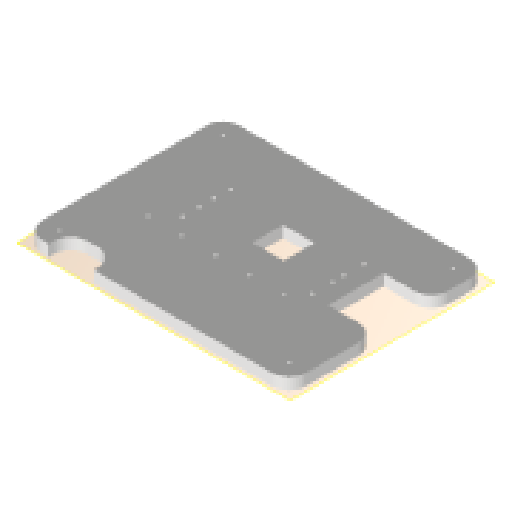
# Autodesk Inventor part: 60_Planktoscope_MicroscopeHolder_Bottom_v0
Saved by Autodesk Inventor 2024.1 (Build 281209000, 209)
## iProperties
Created: 2024-06-29
Part Number: 60_Planktoscope_MicroscopeHolder_Bottom_v0
Material: Generisch
Document SubType Name: Modeling
Designer: diederichbenedict
Density: 1 g/cm^3
Appearance: Vorgabe
Author: diederichbenedict
Autodesk Inventor part; units mm, degrees
ref_plane "YZ Plane" through (0, 0, 0) normal (1, 0, 0) x (0, 1, 0)
ref_plane "XZ Plane" through (0, 0, 0) normal (0, 1, 0) x (-1, 0, 0)
ref_plane "XY Plane" through (0, 0, 0) normal (0, 0, 1) x (1, 0, 0)
ref_plane "Arbeitsebene1" through (0, 0, -15) normal (0, 0, 1) x (1, 0, 0)
sketch "Skizze1" plane through (0, 0, -15) normal (0, 0, 1) x (1, 0, 0)
  line L0 (-108.9123, -85.8768) -> (-108, -84.9645) construction
  line L1 (-108, -84.9645) -> (-105.5687, -87.3957) construction
  arc A0 (-105.5687, -87.3957) -> (-101.5, -88) centre (-101.5, -74) ccw construction
  line L2 (-101.5, -88) -> (-95.5, -88) construction
  line L3 (-95.5, -88) -> (-95.5, -75) construction
  arc A1 (-88.5, -68) -> (-95.5, -75) centre (-88.5, -75) ccw construction
  line L4 (-88.5, -68) -> (-62.5, -68) construction
  arc A2 (-55.5, -75) -> (-62.5, -68) centre (-62.5, -75) ccw construction
  line L5 (-55.5, -75) -> (-55.5, -88) construction
  line L6 (-55.5, -88) -> (101.7625, -88) construction
  arc A3 (101.7625, -88) -> (115.5, -74) centre (101.5, -74.0025) ccw construction
  line L7 (115.5, -74) -> (115.5, 74) construction
  arc A4 (115.5, 74) -> (101.7625, 88) centre (101.5, 74.0025) ccw construction
  line L8 (101.7625, 88) -> (-101.5, 88) construction
  arc A5 (-101.5, 88) -> (-115.5, 74) centre (-101.5, 74) ccw construction
  line L9 (-115.5, 74) -> (-115.5, -74) construction
  arc A6 (-115.5, -74) -> (-108.9123, -85.8768) centre (-101.5, -74) ccw construction
  line L10 (101.6984, -82) -> (101.3016, -82) construction
  arc A7 (101.3016, -82) -> (101.6984, -82) centre (101.5, -74.0025) ccw construction
  line L11 (95.5, 73) -> (95.5, 82) construction
  arc A8 (95.5, 73) -> (100.5, 68) centre (100.5, 73) ccw construction
  line L12 (109.5, 68) -> (100.5, 68) construction
  line L13 (109.5, 68) -> (109.5, -68) construction
  line L14 (100.5, -68) -> (109.5, -68) construction
  arc A9 (100.5, -68) -> (95.5, -73) centre (100.5, -73) ccw construction
  line L15 (95.5, -82) -> (95.5, -73) construction
  line L16 (95.5, -82) -> (-49.5, -82) construction
  line L17 (-49.5, -82) -> (-49.5, -75) construction
  arc A10 (-49.5, -75) -> (-62.5, -62) centre (-62.5, -75) ccw construction
  line L18 (-62.5, -62) -> (-88.5, -62) construction
  arc A11 (-88.5, -62) -> (-99.5163, -68.0977) centre (-88.5, -75) ccw construction
  arc A12 (-99.5163, -68.0977) -> (-100.5, -68) centre (-100.5, -73) ccw construction
  line L19 (-109.5, -68) -> (-100.5, -68) construction
  line L20 (-109.5, -68) -> (-109.5, 68) construction
  line L21 (-100.5, 68) -> (-109.5, 68) construction
  arc A13 (-100.5, 68) -> (-95.5, 73) centre (-100.5, 73) ccw construction
  line L22 (-95.5, 82) -> (-95.5, 73) construction
  line L23 (-95.5, 82) -> (95.5, 82) construction
  arc A14 (101.6984, 82) -> (101.3016, 82) centre (101.5, 74.0025) ccw construction
  line L24 (101.3016, 82) -> (101.6984, 82) construction
  line L25 (111.5331, 80.5) -> (107.9975, 76.9645) construction
  line L26 (107.9975, 76.9645) -> (104.462, 80.5) construction
  line L27 (104.462, 80.5) -> (107.9975, 84.0355) construction
  line L28 (107.9975, 84.0355) -> (111.5331, 80.5) construction
  line L29 (108, -84.0355) -> (104.4645, -80.5) construction
  line L30 (104.4645, -80.5) -> (108, -76.9645) construction
  line L31 (108, -76.9645) -> (111.5355, -80.5) construction
  line L32 (111.5355, -80.5) -> (108, -84.0355) construction
  line L33 (-108, 76.9645) -> (-111.5355, 80.5) construction
  line L34 (-111.5355, 80.5) -> (-108, 84.0355) construction
  line L35 (-108, 84.0355) -> (-104.4645, 80.5) construction
  line L36 (-104.4645, 80.5) -> (-108, 76.9645) construction
  circle A15 centre (58.5, 18.7) radius 1.4 projected
  circle A16 centre (58.5, 36.552) radius 1.4 projected
  circle A17 centre (-57.5, 20.252) radius 1.4 projected
  circle A18 centre (-57.5, 35) radius 1.4 projected
  line L37 (-60.5, 13.7) -> (-60.5, 38) construction
  line L38 (61.5, 13.7) -> (-60.5, 13.7) construction
  line L39 (61.5, 38) -> (61.5, 13.7) construction
  line L40 (61.5, 38) -> (-60.5, 38) construction
  circle A19 centre (58.5, 8.7) radius 1.4 projected
  circle A20 centre (58.5, -9.152) radius 1.4 projected
  circle A21 centre (-57.5, 7.148) radius 1.4 projected
  circle A22 centre (-57.5, -7.6) radius 1.4 projected
  line L41 (-60.5, 13.7) -> (-60.5, -10.6) construction
  line L42 (61.5, -10.6) -> (-60.5, -10.6) construction
  line L43 (61.5, -10.6) -> (61.5, 13.7) construction
  line L44 (61.5, 13.7) -> (-60.5, 13.7) construction
  line L45 (-101.5, 87.5) -> (101.5, 87.5)
  line L46 (116.5, 72.5) -> (116.5, -72.3481)
  line L47 (101.5, -87.3481) -> (-101.5, -87.3481)
  line L48 (-116.5, -72.3481) -> (-116.5, 72.5)
  arc A23 (-116.5, -72.3481) -> (-101.5, -87.3481) centre (-101.5, -72.3481) ccw
  arc A24 (-101.5, 87.5) -> (-116.5, 72.5) centre (-101.5, 72.5) ccw
  arc A25 (116.5, 72.5) -> (101.5, 87.5) centre (101.5, 72.5) ccw
  arc A26 (101.5, -87.3481) -> (116.5, -72.3481) centre (101.5, -72.3481) ccw
  line L49 (-95.5, -88) -> (-56.1, -88)
  line L50 (-56.1, -88) -> (-56.1, -83)
  line L51 (-71.1, -68) -> (-80.5, -68)
  line L52 (-95.5, -83) -> (-95.5, -88)
  arc A27 (-80.5, -68) -> (-95.5, -83) centre (-80.5, -83) ccw
  arc A28 (-56.1, -83) -> (-71.1, -68) centre (-71.1, -83) ccw
  point P0 (0, 0)
  point P1 (-103.5567, -87.8481)
  point P2 (-95.5, -87.3481)
  point P3 (-56.1, -87.3481)
  dimension "d0" = 1
  dimension "d1" = 1
  dimension "d2" = 0.5
  dimension "d3" = 0.5
  dimension "d4" = 15
  dimension "d5" = 15
  constraints: 16 end point, 13 point on circle, 12 tangent, 6 centre point, 4 equal radius, 4 parallel, 2 horizontal, 2 perpendicular
  measures "d0" distance between parallel lines of L48 L9
  measures "d1" distance between parallel lines of L7 L46
  measures "d2" distance between parallel lines of L45 L8
  measures "d3" distance from line of point (-103.557, -87.848) L47
  measures "d4" radius of A23
  measures "d5" radius of A27
extrude "Extrusion1" add sketch "Skizze1" along normal blind 10 draft -1 contours L45 A25 L46 A26 L47 L50 A28 L51 A27 L52 A23 L48 A24
sketch "Skizze3" plane through (0, 0, -5) normal (0, 0, 1) x (1, 0, 0)
  line L0 (116.3254, 72.5) -> (116.3254, -72.3481) projected
  arc A0 (116.3254, 72.5) -> (101.5, 87.3254) centre (101.5, 72.5) ccw projected
  line L1 (-101.5, 87.3254) -> (101.5, 87.3254) projected
  arc A1 (-101.5, 87.3254) -> (-116.3254, 72.5) centre (-101.5, 72.5) ccw projected
  line L2 (-116.3254, -72.3481) -> (-116.3254, 72.5) projected
  arc A2 (-116.3254, -72.3481) -> (-101.5, -87.1736) centre (-101.5, -72.3481) ccw projected
  line L3 (-95.6746, -87.1736) -> (-101.5, -87.1736) projected
  line L4 (-95.6746, -83) -> (-95.6746, -87.1736) projected
  arc A3 (-80.5, -67.8254) -> (-95.6746, -83) centre (-80.5, -83) ccw projected
  line L5 (-71.1, -67.8254) -> (-80.5, -67.8254) projected
  arc A4 (-55.9254, -83) -> (-71.1, -67.8254) centre (-71.1, -83) ccw projected
  line L6 (-55.9254, -87.1736) -> (-55.9254, -83) projected
  line L7 (101.5, -87.1736) -> (-55.9254, -87.1736) projected
  arc A5 (101.5, -87.1736) -> (116.3254, -72.3481) centre (101.5, -72.3481) ccw projected
  circle A6 centre (58.5, 18.7) radius 1.5746 projected
  circle A7 centre (58.5, 36.552) radius 1.5746 projected
  circle A8 centre (-57.5, 20.252) radius 1.5746 projected
  circle A9 centre (-57.5, 35) radius 1.5746 projected
  circle A10 centre (58.5, 8.7) radius 1.5746 projected
  circle A11 centre (58.5, -9.152) radius 1.5746 projected
  circle A12 centre (-57.5, 7.148) radius 1.5746 projected
  circle A13 centre (-57.5, -7.6) radius 1.5746 projected
  point P0 (0, 0)
hole "Bohrung1" at (-101.5, 72.5, -5) at (-101.5, -72.3481, -5) at (101.5, -72.3481, -5) at (101.5, 72.5, -5) direction (0, 0, -1) diameter 2.8 end through all
sketch "Skizze4" plane through (0, 0, -5) normal (0, 0, 1) x (1, 0, 0)
  line L0 (-2.75, 38) -> (-2.75, 23.7) projected
  line L1 (-6.0553, 13.7) -> (-6.0553, 30)
  line L2 (20.9, 30.6837) -> (20.9, 6.6837) projected
  line L3 (20.9, 30.6837) -> (-6.8742, 30.6837)
  line L4 (-6.8742, 30.6837) -> (-6.8742, 3.5446)
  line L5 (-6.8742, 3.5446) -> (20.9, 3.5446)
  line L6 (20.9, 3.5446) -> (20.9, 30.6837)
  point P0 (0, 0)
  constraints: 10 end point, 2 parallel, 1 horizontal, 1 perpendicular, 1 vertical, 2 other
extrude "Extrusion3" cut sketch "Skizze4" against normal through all
sketch "Skizze5" plane through (0, 0, -5) normal (0, 0, 1) x (1, 0, 0)
  line L0 (-6.8742, 30.6837) -> (20.9, 30.6837) projected
  line L1 (20.9, 30.6837) -> (20.9, 3.5446) projected
  line L2 (20.9, 3.5446) -> (-6.8742, 3.5446) projected
  line L3 (-6.8742, 3.5446) -> (-6.8742, 30.6837) projected
  circle A0 centre (101.5, 72.5) radius 1.4 projected
  circle A1 centre (101.5, -72.3481) radius 1.4 projected
  circle A2 centre (-101.5, -72.3481) radius 1.4 projected
  circle A3 centre (-101.5, 72.5) radius 1.4 projected
  line L4 (116.3254, 72.5) -> (116.3254, -72.3481) projected
  arc A4 (116.3254, 72.5) -> (101.5, 87.3254) centre (101.5, 72.5) ccw projected
  line L5 (-101.5, 87.3254) -> (101.5, 87.3254) projected
  arc A5 (-101.5, 87.3254) -> (-116.3254, 72.5) centre (-101.5, 72.5) ccw projected
  line L6 (-116.3254, -72.3481) -> (-116.3254, 72.5) projected
  arc A6 (-116.3254, -72.3481) -> (-101.5, -87.1736) centre (-101.5, -72.3481) ccw projected
  line L7 (-95.6746, -87.1736) -> (-101.5, -87.1736) projected
  line L8 (-95.6746, -83) -> (-95.6746, -87.1736) projected
  arc A7 (-80.5, -67.8254) -> (-95.6746, -83) centre (-80.5, -83) ccw projected
  line L9 (-71.1, -67.8254) -> (-80.5, -67.8254) projected
  arc A8 (-55.9254, -83) -> (-71.1, -67.8254) centre (-71.1, -83) ccw projected
  line L10 (-55.9254, -87.1736) -> (-55.9254, -83) projected
  line L11 (101.5, -87.1736) -> (-55.9254, -87.1736) projected
  arc A9 (101.5, -87.1736) -> (116.3254, -72.3481) centre (101.5, -72.3481) ccw projected
  circle A10 centre (58.5, 18.7) radius 1.5746 projected
  circle A11 centre (58.5, 36.552) radius 1.5746 projected
  circle A12 centre (-57.5, 20.252) radius 1.5746 projected
  circle A13 centre (-57.5, 35) radius 1.5746 projected
  circle A14 centre (58.5, 8.7) radius 1.5746 projected
  circle A15 centre (58.5, -9.152) radius 1.5746 projected
  circle A16 centre (-57.5, 7.148) radius 1.5746 projected
  circle A17 centre (-57.5, -7.6) radius 1.5746 projected
  line L12 (-73.1917, -22.4328) -> (70.9104, -22.4328)
  line L13 (102.338, 36.5746) -> (102.338, -9.1746)
  point P0 (0, 0)
  point P1 (-43.1917, -22.4328)
  point P2 (-13.1917, -22.4328)
  point P3 (16.8083, -22.4328)
  point P4 (46.8083, -22.4328)
  point P5 (102.338, 13.7)
  point P6 (102.338, -1.3)
  point P7 (102.338, 28.7)
  point P8 (102.338, 13.7)
  dimension "d21" = 30
  dimension "d36" = 15
  dimension "d39" = 15
  constraints: 4 end point, 3 vertical, 2 horizontal, 1 coincident, 1 midpoint, 7 other
  measures "d21" distance of point (-73.192, -22.433) point (-43.192, -22.433)
  measures "d36" distance of point (102.338, 13.7) point (102.338, -1.3)
  measures "d39" distance of point (102.338, 13.7) point (102.338, 28.7)
hole "Bohrung2" at (-73.1917, -22.4328, -5) at (-43.1917, -22.4328, -5) at (-13.1917, -22.4328, -5) at (16.8083, -22.4328, -5) at (46.8083, -22.4328, -5) at (102.338, -1.3, -5) at (102.338, 13.7, -5) at (102.338, 28.7, -5) direction (0, 0, -1) diameter 2.8 end through all
